Autodesk Fusion 360 part; units mm, degrees
(part 2 of 2)
component "old_component (4)" placed x (0.34757, 0.936466, 0.047176) y (-0.741638, 0.305348, -0.597273) z (-0.573731, 0.172607, 0.800649) at (269.6365, 81.223, -924.0278)
component "old_component (5)" placed x (0.34757, 0.936466, 0.047176) y (-0.741638, 0.305348, -0.597273) z (-0.573731, 0.172607, 0.800649) at (327.5833, 63.7897, -1004.8934)
component "old_component (6)" placed x (0.71799, 0.576369, 0.390243) y (-0.394111, 0.798753, -0.454611) z (-0.573731, 0.172607, 0.800649) at (533.2687, 130.1276, -1120.3526)
component "old_component (7)" placed x (0.71799, 0.576369, 0.390243) y (0.69493, -0.561735, -0.448916) z (-0.039528, 0.593509, -0.803856) at (-2006.1716, -2376.8812, 7254.5735)
component "old_component (8)" placed x (-0.791305, 0.472641, 0.387875) y (0.610143, 0.651427, 0.450964) z (-0.039528, 0.593509, -0.803856) at (-2075.3249, -2103.5181, 7459.8054)
component "old_component (9)" placed x (0.66668, -0.729674, 0.152031) y (-0.610143, -0.651427, -0.450964) z (0.428094, 0.207888, -0.879499) at (-4981.8989, -279.6575, 7657.1742)
component "old_component (10)" placed x (0.413097, 0.224133, -0.882675) y (-0.610143, -0.651427, -0.450964) z (-0.676075, 0.724849, -0.13235) at (1312.0652, -3188.2376, 3343.111)
component "old_component (11)" placed x (0.008638, 0.563686, -0.825944) y (-0.610143, -0.651427, -0.450964) z (-0.792245, 0.507839, 0.338302) at (1839.4358, -1946.8039, 836.3127)
component "old_component (12)" placed x (0.351588, -0.732695, 0.582704) y (-0.610143, -0.651427, -0.450964) z (0.710008, -0.196979, -0.676083) at (-6490.517, 1910.2312, 6534.9519)
component "old_component (13)" placed x (0.999418, 0.01979, -0.027799) y (-0.019053, 0.999466, 0.026549) z (0.02831, -0.026004, 0.999261) at (-66.1814, 125.0503, -91.0962)
component "old_component (14)" placed x (0.999563, -0.016547, 0.024494) y (0.017101, 0.999599, -0.022558) z (-0.024111, 0.022967, 0.999445) at (55.8203, -107.4599, 79.7048)
component "Component2_1" placed x (1, 0, 0) y (0, 1, 0) z (0, 0, 1) at (0, 0, 0)
component "Component3_1" placed x (1, 0, 0) y (0, 1, 0) z (0, 0, 1) at (0, 0, 0)
component "base_link" placed x (1, 0, 0) y (0, 1, 0) z (0, 0, 1) at (0, 0, 0)
component "Component5_1" placed x (1, 0, 0) y (0, 1, 0) z (0, 0, 1) at (0, 0, 0)
component "Component6_1" placed x (1, 0, 0) y (0, 1, 0) z (0, 0, 1) at (0, 0, 0)
component "Component7_1" placed x (1, 0, 0) y (0, 1, 0) z (0, 0, 1) at (0, 0, 0)
component "Component8_1" placed x (1, 0, 0) y (0, 1, 0) z (0, 0, 1) at (0, 0, 0)
component "Component9_1" placed x (1, 0, 0) y (0, 1, 0) z (0, 0, 1) at (0, 0, 0)
component "Component10_1" placed x (1, 0, 0) y (0, 1, 0) z (0, 0, 1) at (0, 0, 0)
component "Component11_1" placed x (1, 0, 0) y (0, 1, 0) z (0, 0, 1) at (0, 0, 0)
component "Component12_1" placed x (1, 0, 0) y (0, 1, 0) z (0, 0, 1) at (0, 0, 0)
component "Component13_1" placed x (1, 0, 0) y (0, 1, 0) z (0, 0, 1) at (0, 0, 0)
component "Component14_1" placed x (1, 0, 0) y (0, 1, 0) z (0, 0, 1) at (0, 0, 0)
component "Component15_1" placed x (1, 0, 0) y (0, 1, 0) z (0, 0, 1) at (0, 0, 0)
component "Component16_1" placed x (1, 0, 0) y (0, 1, 0) z (0, 0, 1) at (0, 0, 0)
